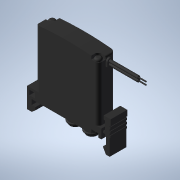
# Autodesk Inventor part: SX12F-KH
Saved by Autodesk Inventor 2024.3 (Build 283343000, 343)
## iProperties
Category: PARTsolutions
Company: SMC
Created: 2025-06-09
Part Number: SX12F-KH
Material: Generic
Catalog Web Link: www.cadenas.de
Description: SX10-High Speed 2 Port Valve
Vendor: SMC
Document SubType Name: Modeling
Designer: psAdmin
Manufacturer: SMC
Mass: 12.0949 g
Surface Area: 51.7491 cm^2
Volume: 12.0949 cm^3
Density: 1 g/cm^3
Appearance: PSOLRGB-175-175-175
PSOL_IDENT_0: {$CADENAS_DATA/23d-libs/smc/fluid_control_equipment/process_valves/air_blows/sx10/sx10.prj},177 {VTY
PSOL_IDENT_1: P=3D},{NB=SX12F-KH},{LINA=SX12F-KH},{NN=SX10},{DATE=22.05.2025 10:26:26},{GEOMDATE=14.05.2014 05:43:
PSOL_IDENT_2: 46},{VERSION=},{LINEID=10},{WBVAR=MOUNT,FILTER,FRAOF,LEAD},{WBNUMERIC=}  {NB=SX12F-KH},{LINA=SX12F-K
PSOL_IDENT_3: H},{KT=DUMMY},{ORDER=SX12F-KH},{MOUNT=2},{FILTER=F},{FRAOF=K},{LEAD=H},{MODEL=SX12F-KH}
NB: SX12F-KH
NN: SX10
NT: High Speed 2 Port Valve
NBSYN: $ORDER.
LINA: SX12F-KH
CATALOG: SMC
MOUNT: (2) Quick disconnect type
FILTER: (F) With filter
FRAOF: (K) Flow rate 150 L/min, Max. operating frequency 500 Hz
LEAD: (H) 500 mm
SUPPLIER: SMC
ARTICLENO: SX12F-KH
BOMINFO: SX12F-KH
CREATOR: CADENAS GmbH
Title: SX12F-KH
Author: Cadenas PARTsolutions
Comments: High Speed 2 Port Valve
Autodesk Inventor part; units mm, degrees
ref_plane "YZ Plane" through (0, 0, 0) normal (1, 0, 0) x (0, 1, 0)
ref_plane "XZ Plane" through (0, 0, 0) normal (0, 1, 0) x (-1, 0, 0)
ref_plane "XY Plane" through (0, 0, 0) normal (0, 0, 1) x (1, 0, 0)
sketch "Sketch_7" plane through (0, 0, 0) normal (0, 0, 1) x (1, 0, 0)
  line L0 (-21.5, -5.9) -> (-19, -5.9)
  line L1 (-19, -5.9) -> (-17, -4.2218)
  line L2 (-17, -4.2218) -> (-17, -2.7)
  line L3 (-17, -2.7) -> (-19, -2.7)
  line L4 (-19, -2.7) -> (-19, 0)
  line L5 (-19, 0) -> (18.5, 0)
  line L6 (18.5, 0) -> (18.5, 2.5)
  line L7 (18.5, 2.5) -> (21, 2.5)
  line L8 (21, 2.5) -> (21, -2.7)
  line L9 (21, -2.7) -> (19.5, -2.7)
  line L10 (19.5, -2.7) -> (19.5, -3.1939)
  line L11 (19.5, -3.1939) -> (21, -5.9)
  line L12 (21, -5.9) -> (23, -5.9)
  line L13 (23, -5.9) -> (23, 3)
  line L14 (23, 3) -> (23.3, 3)
  line L15 (23.3, 3) -> (23.3, 4)
  line L16 (23.3, 4) -> (23, 4)
  line L17 (23, 4) -> (23, 5)
  line L18 (23, 5) -> (23.3, 5)
  line L19 (23.3, 5) -> (23.3, 6)
  line L20 (23.3, 6) -> (23, 6)
  line L21 (23, 6) -> (23, 7)
  line L22 (23, 7) -> (23.3, 7)
  line L23 (23.3, 7) -> (23.3, 8)
  line L24 (23.3, 8) -> (23, 8)
  line L25 (23, 8) -> (23, 8.3)
  line L26 (23, 8.3) -> (23.5, 8.8)
  line L27 (23.5, 8.8) -> (23.5, 11.8)
  line L28 (23.5, 11.8) -> (19.75, 11.8)
  line L29 (19.75, 11.8) -> (19.75, 9.8)
  line L30 (19.75, 9.8) -> (20.55, 9.8)
  line L31 (20.55, 9.8) -> (20.55, 3.5)
  line L32 (20.55, 3.5) -> (18.5, 3.5)
  line L33 (18.5, 3.5) -> (18.5, 5)
  line L34 (18.5, 5) -> (-21.5, 5)
  line L35 (-21.5, 5) -> (-21.5, -5.9)
  line L36 (-20.3, 3.8) -> (-20.3, 1.2)
  line L37 (-20.3, 1.2) -> (-17.2, 1.2)
  line L38 (-17.2, 1.2) -> (-17.2, 3.8)
  line L39 (-17.2, 3.8) -> (-20.3, 3.8)
  constraints: 80 end point
extrude "Extrusion1" add sketch "Sketch_7" along normal mid plane 9
sketch "Sketch_2" plane through (0, 5, 0) normal (0, 1, 0) x (1, 0, 0)
  line L0 (-17, 2.5) -> (-17, -2.5)
  arc A0 (-17, -2.5) -> (-15, -4.5) centre (-15, -2.5) ccw
  line L1 (-15, -4.5) -> (15, -4.5)
  arc A1 (15, -4.5) -> (17, -2.5) centre (15, -2.5) ccw
  line L2 (17, -2.5) -> (17, 2.5)
  arc A2 (17, 2.5) -> (15, 4.5) centre (15, 2.5) ccw
  line L3 (15, 4.5) -> (-15, 4.5)
  arc A3 (-15, 4.5) -> (-17, 2.5) centre (-15, 2.5) ccw
  constraints: 8 end point, 8 point on circle, 4 centre point
extrude "Extrusion2" add sketch "Sketch_2" along normal blind 31.9
sketch "Sketch_3" plane through (0, 0, 0) normal (0, 0, 1) x (1, 0, 0)
  line L0 (-19, 41) -> (-19, 6)
  line L1 (-19, 6) -> (-17, 6)
  line L2 (-17, 6) -> (-17, 35.2179)
  arc A0 (-16.2869, 36.0132) -> (-17, 35.2179) centre (-16.2, 35.2179) ccw
  arc A1 (16.2869, 36.0132) -> (-16.2869, 36.0132) centre (0, -113.1) ccw
  arc A2 (17, 35.2179) -> (16.2869, 36.0132) centre (16.2, 35.2179) ccw
  line L3 (17, 35.2179) -> (17, 6)
  line L4 (17, 6) -> (19, 6)
  line L5 (19, 6) -> (19, 41)
  line L6 (19, 41) -> (-19, 41)
  constraints: 14 end point, 6 point on circle, 3 centre point
extrude "Extrusion3" cut sketch "Sketch_3" along normal mid plane 9
sketch "Sketch_4" plane through (0, 34.53, 0) normal (0, 1, 0) x (1, 0, 0)
  line L0 (13.05, -4.5) -> (17, -4.5)
  line L1 (17, -4.5) -> (17, -0.6)
  line L2 (17, -0.6) -> (14.95, -0.6)
  arc A0 (14.95, -0.6) -> (13.05, -2.5) centre (14.95, -2.5) ccw
  line L3 (13.05, -2.5) -> (13.05, -4.5)
  constraints: 8 end point, 2 point on circle, 1 centre point
extrude "Extrusion4" cut sketch "Sketch_4" along normal blind 3
sketch "Sketch_5" plane through (0, 34.53, 0) normal (0, 1, 0) x (1, 0, 0)
  line L0 (-17, 4.5) -> (-17, 0.6)
  line L1 (-17, 0.6) -> (-14.95, 0.6)
  arc A0 (-14.95, 0.6) -> (-13.05, 2.5) centre (-14.95, 2.5) ccw
  line L2 (-13.05, 2.5) -> (-13.05, 4.5)
  line L3 (-13.05, 4.5) -> (-17, 4.5)
  constraints: 8 end point, 2 point on circle, 1 centre point
extrude "Extrusion5" cut sketch "Sketch_5" along normal blind 4.5
sketch "Sketch_6" plane through (18.5, 3.5, -4.5) normal (0, 1, 0) x (1, 0, 0)
  line L0 (0, 0) -> (0, -1)
  line L1 (0, -1) -> (2.05, -1)
  line L2 (2.05, -1) -> (2.05, 0)
  line L3 (2.05, 0) -> (0, 0)
  constraints: 8 end point
extrude "Extrusion6" cut sketch "Sketch_6" against normal blind 1
sketch "Sketch_8" plane through (20.55, 3.5, 4.5) normal (0, 1, 0) x (-1, 0, 0)
  line L0 (0, -1) -> (2.05, -1)
  line L1 (2.05, -1) -> (2.05, 0)
  line L2 (2.05, 0) -> (0, 0)
  line L3 (0, 0) -> (0, -1)
  constraints: 8 end point
extrude "Extrusion7" cut sketch "Sketch_8" against normal blind 1
sketch "Sketch_9" plane through (0, 0, 2.5) normal (0, 0, 1) x (1, 0, 0)
  line L0 (14.95, 34.53) -> (14.95, 35.83)
  line L1 (14.95, 35.83) -> (15.7, 35.83)
  arc A0 (16.7, 34.83) -> (15.7, 35.83) centre (15.7, 34.83) ccw
  line L2 (16.7, 34.83) -> (16.7, 34.53)
  line L3 (16.7, 34.53) -> (14.95, 34.53)
  line L4 (14.95, 34.53) -> (14.95, 35.83)
  constraints: 10 end point, 2 point on circle, 1 centre point
revolve "Revolution1" add sketch "Sketch_9" angle 360 about axis through (14.95, 34.53, 2.5) along (0, -1, 0)
sketch "Sketch_10" plane through (0, 0, -2.5) normal (0, 0, 1) x (1, 0, 0)
  line L0 (-14.95, 34.53) -> (-14.95, 35.83)
  line L1 (-14.95, 35.83) -> (-14.2, 35.83)
  arc A0 (-13.2, 34.83) -> (-14.2, 35.83) centre (-14.2, 34.83) ccw
  line L2 (-13.2, 34.83) -> (-13.2, 34.53)
  line L3 (-13.2, 34.53) -> (-14.95, 34.53)
  line L4 (-14.95, 34.53) -> (-14.95, 35.83)
  constraints: 10 end point, 2 point on circle, 1 centre point
revolve "Revolution2" add sketch "Sketch_10" angle 360 about axis through (-14.95, 34.53, -2.5) along (0, -1, 0)
sketch "Sketch_19" plane through (17, 0, 0) normal (1, 0, 0) x (0, 0, -1)
  line L0 (-0.5679, 31.23) -> (2.3679, 31.23)
  line L1 (2.3679, 31.23) -> (2.3679, 33.63)
  arc A0 (2.3679, 33.63) -> (-0.5679, 33.63) centre (0.9, 33.63) ccw
  line L2 (-0.5679, 33.63) -> (-0.5679, 31.23)
  constraints: 6 end point, 2 point on circle, 1 centre point
extrude "Extrusion8" add sketch "Sketch_19" along normal blind 0.9
sketch "Sketch_20" plane through (0, 0, -0.9) normal (0, 0, 1) x (1, 0, 0)
  line L0 (17, 32.08) -> (37.32, 32.08)
  line L1 (37.32, 32.08) -> (37.32, 31.76)
  line L2 (37.32, 31.76) -> (33.32, 31.76)
  line L3 (33.32, 31.76) -> (33.32, 31.305)
  line L4 (33.32, 31.305) -> (17, 31.305)
  line L5 (17, 31.305) -> (17, 32.08)
  line L6 (17, 32.08) -> (37.32, 32.08)
  constraints: 14 end point
revolve "Revolution3" add sketch "Sketch_20" angle 360 about axis through (17, 32.08, -0.9) along (-1, 0, 0)
sketch "Sketch_21" plane through (0, 0, -0.9) normal (0, 0, 1) x (1, 0, 0)
  line L0 (17, 33.63) -> (37.32, 33.63)
  line L1 (37.32, 33.63) -> (37.32, 33.31)
  line L2 (37.32, 33.31) -> (33.32, 33.31)
  line L3 (33.32, 33.31) -> (33.32, 32.865)
  line L4 (33.32, 32.865) -> (17, 32.865)
  line L5 (17, 32.865) -> (17, 33.63)
  line L6 (17, 33.63) -> (37.32, 33.63)
  constraints: 14 end point
revolve "Revolution4" add sketch "Sketch_21" angle 360 about axis through (17, 33.63, -0.9) along (-1, 0, 0)
sketch "Sketch_22" plane through (0, 0, 0) normal (0, 1, 0) x (-1, 0, 0)
  arc A0 (16.85, -2.5) -> (13.05, -2.5) centre (14.95, -2.5) ccw
  line L0 (13.05, -2.5) -> (13.05, -4.5)
  line L1 (13.05, -4.5) -> (16.85, -4.5)
  line L2 (16.85, -4.5) -> (16.85, -2.5)
  constraints: 6 end point, 2 point on circle, 1 centre point
extrude "Extrusion9" cut sketch "Sketch_22" along normal blind 2
sketch "Sketch_23" plane through (0, 0, 0) normal (0, 1, 0) x (-1, 0, 0)
  line L0 (-13.05, 2.5) -> (-13.05, 4.5)
  line L1 (-13.05, 4.5) -> (-16.85, 4.5)
  line L2 (-16.85, 4.5) -> (-16.85, 2.5)
  arc A0 (-16.85, 2.5) -> (-13.05, 2.5) centre (-14.95, 2.5) ccw
  constraints: 6 end point, 2 point on circle, 1 centre point
extrude "Extrusion10" cut sketch "Sketch_23" along normal blind 2
sketch "Sketch_24" plane through (0, 0, 2.5) normal (0, 0, 1) x (1, 0, 0)
  line L0 (14.95, 0.7) -> (14.95, 2)
  line L1 (14.95, 2) -> (16.7, 2)
  line L2 (16.7, 2) -> (16.7, 1.7)
  arc A0 (15.7, 0.7) -> (16.7, 1.7) centre (15.7, 1.7) ccw
  line L3 (15.7, 0.7) -> (14.95, 0.7)
  line L4 (14.95, 0.7) -> (14.95, 2)
  constraints: 10 end point, 2 point on circle, 1 centre point
revolve "Revolution5" add sketch "Sketch_24" angle 360 about axis through (14.95, 0.7, 2.5) along (0, -1, 0)
sketch "Sketch_25" plane through (0, 0, -2.5) normal (0, 0, 1) x (1, 0, 0)
  line L0 (-14.95, 0.7) -> (-14.95, 2)
  line L1 (-14.95, 2) -> (-13.2, 2)
  line L2 (-13.2, 2) -> (-13.2, 1.7)
  arc A0 (-14.2, 0.7) -> (-13.2, 1.7) centre (-14.2, 1.7) ccw
  line L3 (-14.2, 0.7) -> (-14.95, 0.7)
  line L4 (-14.95, 0.7) -> (-14.95, 2)
  constraints: 10 end point, 2 point on circle, 1 centre point
revolve "Revolution6" add sketch "Sketch_25" angle 360 about axis through (-14.95, 0.7, -2.5) along (0, -1, 0)
sketch "Sketch_26" plane through (0, 0, 0) normal (0, 0, 1) x (1, 0, 0)
  line L0 (0, -3.8) -> (0, 0)
  line L1 (1.9, 0) -> (1.9, -3.8)
  line L2 (1.9, -3.8) -> (2.8113, -3.8)
  line L3 (2.8113, -3.8) -> (3.1, -3.3)
  line L4 (3.1, -3.3) -> (3.1, -2.8)
  line L5 (3.1, -2.8) -> (2.8, -2.8)
  arc A0 (2.6677, -2.75) -> (2.8, -2.8) centre (2.8, -2.6) ccw
  line L6 (2.6677, -2.75) -> (3.2, -2.75)
  arc A1 (3.2, -2.75) -> (3.2, -1.55) centre (3.2, -2.15) ccw
  line L7 (3.2, -1.55) -> (2.6677, -1.55)
  arc A2 (2.8, -1.5) -> (2.6677, -1.55) centre (2.8, -1.7) ccw
  line L8 (2.8, -1.5) -> (3.45, -1.5)
  line L9 (3.45, -1.5) -> (3.45, 0)
  line L10 (3.45, 0) -> (1.9, 0)
  constraints: 22 end point, 6 point on circle, 3 centre point
revolve "Revolution7" add sketch "Sketch_26" angle 360 about axis through (0, -3.8, 0) along (0, -1, 0)
sketch "Sketch_27" plane through (0, 0, 0) normal (0, 0, 1) x (1, 0, 0)
  line L0 (9, -3.8) -> (9, 0)
  line L1 (10.9, 0) -> (10.9, -3.8)
  line L2 (10.9, -3.8) -> (11.8113, -3.8)
  line L3 (11.8113, -3.8) -> (12.1, -3.3)
  line L4 (12.1, -3.3) -> (12.1, -2.8)
  line L5 (12.1, -2.8) -> (11.8, -2.8)
  arc A0 (11.6677, -2.75) -> (11.8, -2.8) centre (11.8, -2.6) ccw
  line L6 (11.6677, -2.75) -> (12.2, -2.75)
  arc A1 (12.2, -2.75) -> (12.2, -1.55) centre (12.2, -2.15) ccw
  line L7 (12.2, -1.55) -> (11.6677, -1.55)
  arc A2 (11.8, -1.5) -> (11.6677, -1.55) centre (11.8, -1.7) ccw
  line L8 (11.8, -1.5) -> (12.45, -1.5)
  line L9 (12.45, -1.5) -> (12.45, 0)
  line L10 (12.45, 0) -> (10.9, 0)
  constraints: 22 end point, 6 point on circle, 3 centre point
revolve "Revolution8" add sketch "Sketch_27" angle 360 about axis through (9, -3.8, 0) along (0, -1, 0)
body "Solid1"
